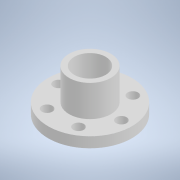
# Autodesk Inventor part: Leo-Berman-Section-Part-3
Saved by Autodesk Inventor 2022 (Build 260153000, 153)
## iProperties
Created: 2022-03-23
Part Number: Leo-Berman-Section-Part-3
Material: Generic
Document SubType Name: Modeling
Designer: leogr
Density: 1 g/cm^3
Appearance: Default
Author: leogr
Autodesk Inventor part; units mm, degrees
ref_plane "YZ Plane" through (0, 0, 0) normal (1, 0, 0) x (0, 1, 0)
ref_plane "XZ Plane" through (0, 0, 0) normal (0, 1, 0) x (-1, 0, 0)
ref_plane "XY Plane" through (0, 0, 0) normal (0, 0, 1) x (1, 0, 0)
sketch "Sketch1" plane through (0, 0, 0) normal (0, 1, 0) x (-1, 0, 0)
  circle A0 centre (0, 0) radius 101.6
  circle A1 centre (0, 0) radius 76.2
  circle A2 centre (76.2, 0) radius 12.7
  circle A3 centre (38.1, 65.9911) radius 12.7
  circle A4 centre (-38.1, 65.9911) radius 12.7
  circle A5 centre (-76.2, 0) radius 12.7
  circle A6 centre (-38.1, -65.9911) radius 12.7
  circle A7 centre (38.1, -65.9911) radius 12.7
  circle A8 centre (0, 0) radius 38.1
  dimension "d1" = 152.4
  dimension "d0" = 203.2
  dimension "d2" = 25.4
  dimension "d5" = 360
  dimension "d7" = 76.2
  constraints: 8 centre point, 3 coincident, 1 horizontal alignment, 15 other
  measures "d0" diameter of A0
  measures "d2" diameter of A2
  measures "d7" diameter of A8
extrude "Extrusion1" add sketch "Sketch1" along normal mid plane 25.4 contours A0 | A2 A1 A7 A6 A5 A4 A3
sketch "Sketch2" plane through (0, 12.7, 0) normal (0, 1, 0) x (1, 0, 0)
  circle A0 centre (0, 0) radius 38.1 projected
  circle A1 centre (0, 0) radius 50.8
  dimension "d10" = 101.6
  constraints: 1 centre point, 1 coincident
  measures "d10" diameter of A1
extrude "Extrusion2" add sketch "Sketch2" along normal blind 76.2
body "Solid1"
